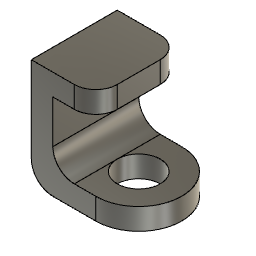
Exercise_03 (Autodesk Fusion 360 design; units mm, degrees)
Autodesk Fusion 360 part; units mm, degrees
note: some values were not read from the file. Set by a fixed rule: which sketch regions a step uses.
sketch "Sketch1" plane through (0, 0, 0) normal (0, 0, 1) x (1, 0, 0)
  circle A0 centre (0, 0) radius 20
  circle A1 centre (0, 0) radius 10
  line L0 (0, 20) -> (-30, 20)
  line L1 (-30, 20) -> (-30, -20)
  line L2 (-30, -20) -> (0, -20)
  line L3 (0, -20) -> (0, 20)
  dimension "d1" = 40
  dimension "d2" = 20
  dimension "d3" = 30
  dimension "d4" = 40
  constraint coincident A0.centre A1.centre
  constraint horizontal L0
  constraint vertical L1
  constraint horizontal L2
  constraint vertical L3
  constraint coincident A0 L0.start
  measures "d1" diameter of A0
  measures "d2" diameter of A1
  measures "d3" distance of L0.start L0.end
  measures "d4" distance of L0.start L2.end
extrude "Extrude1" add sketch "Sketch1" along normal blind 10 contours A0 A1 L3 | A0 A1 L3 | A0 L0 L1 L2
sketch "Sketch2" plane through (0, -20, 0) normal (0, -1, 0) x (1, 0, 0)
  line L0 (-30, 0) -> (0, 0)
  line L1 (0, 0) -> (0, 10)
  line L2 (0, 10) -> (-30, 10)
  line L3 (-30, 10) -> (-30, 0)
  line L4 (-30, 0) -> (-20, 0)
  line L5 (-20, 0) -> (-20, 50.06)
  line L6 (-20, 50.06) -> (-30, 50.06)
  line L7 (-30, 50.06) -> (-30, 0)
  dimension "d7" = 10
  dimension "d8" = 50.06
  constraint horizontal L4
  constraint vertical L5
  constraint horizontal L6
  constraint vertical L7
  constraint coincident L0.start L3.end
  measures "d7" distance of L0.start L4.end
  measures "d8" distance of L0.start L6.end
extrude "Extrude2" add sketch "Sketch2" against normal blind 40 contours L2 L5 L6 L7
fillet "Fillet1" radius 10 1 edges at (-30, 0, 0)
fillet "Fillet2" radius 10 1 edges at (-20, 0, 10)
sketch "Sketch3" plane through (-30, 0, 0) normal (-1, 0, 0) x (0, -1, 0)
  line L0 (-20, 10) -> (20, 10)
  line L1 (20, 10) -> (20, 50.06)
  line L2 (20, 50.06) -> (-20, 50.06)
  line L3 (-20, 50.06) -> (-20, 10)
  line L4 (-20, 50.06) -> (20, 50.06)
  line L5 (20, 50.06) -> (20, 40.06)
  line L6 (20, 40.06) -> (-20, 40.06)
  line L7 (-20, 40.06) -> (-20, 50.06)
  dimension "d15" = 10
  constraint horizontal L4
  constraint vertical L5
  constraint horizontal L6
  constraint vertical L7
  constraint coincident L2.end L3.start
  measures "d15" distance of L2.end L6.end
extrude "Extrude3" add sketch "Sketch3" against normal blind 30 contours L1 L2 L3 L4 L5 L6 L7
fillet "Fillet3" radius 10 2 edges at (0, 20, 45.06) (0, -20, 45.06)
